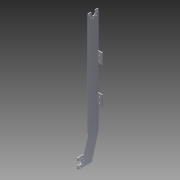
# Autodesk Inventor part: 09
Saved by Autodesk Inventor 2013 (Build 170138000, 138)
## iProperties
Created: 2014-03-10
Part Number: 09
Material: アルミニウム 6061
Document SubType Name: Modeling
Designer: andou
Density: 1 g/cm^3
Author: andou
Title: Dual_Link_Flame(right)
Autodesk Inventor part; units mm, degrees
ref_plane "YZ Plane" through (0, 0, 0) normal (1, 0, 0) x (0, 1, 0)
ref_plane "XZ Plane" through (0, 0, 0) normal (0, 1, 0) x (-1, 0, 0)
ref_plane "XY Plane" through (0, 0, 0) normal (0, 0, 1) x (1, 0, 0)
sketch "スケッチ1" plane through (0, 0, 0) normal (1, 0, 0) x (0, 1, 0)
  line L0 (-20, 125) -> (20, 125)
  line L1 (20, 125) -> (20, -125)
  line L2 (20, -125) -> (-20, -125)
  line L3 (-20, -125) -> (-20, 125)
  point P0 (0, 0)
  dimension "d0" = 250
  dimension "d2" = 40
  dimension "d3" = 20
  dimension "d4" = 125
  constraints: 8 end point, 2 parallel, 1 horizontal, 1 perpendicular
  measures "d0" distance of L2.end L0.start
  measures "d2" distance of L1.end L2.end
  measures "d3" distance from line of L3 point (0, 0)
  measures "d4" distance from line of point (0, 0) L2
extrude "押し出し1" add sketch "スケッチ1" along normal blind 2
sketch "スケッチ3" plane through (0, 0, 0) normal (-1, 0, 0) x (0, 0, 1)
  line L0 (125, -20) -> (125, 20) projected
  line L1 (125, 20) -> (-125, 20) projected
  line L2 (-125, 20) -> (-125, -20) projected
  line L3 (-125, -20) -> (125, -20) projected
  line L4 (-105, -20) -> (-105, -8.0385)
  line L5 (-105, -8.0385) -> (-75, 0)
  line L6 (-75, 0) -> (125, 0)
  line L7 (125, 0) -> (125, 20)
  line L8 (-125, 6.6025) -> (-75, 20)
  point P0 (0, 0)
  dimension "d11" = 20
  dimension "d12" = 15
  dimension "d13" = 15
  dimension "d14" = 20
  dimension "d15" = 250
  dimension "d17" = 200
  dimension "d18" = 200
  constraints: 10 end point, 4 point on line, 3 perpendicular
  measures "d11" distance between parallel lines of L2 L4
  measures "d12" angle of L1 L8
  measures "d13" angle of L6 L5
  measures "d14" distance between parallel lines of L1 L6
  measures "d15" distance between parallel lines of L2 L7
  measures "d17" distance of L7.end L8.end
  measures "d18" distance of L6.end L5.end
extrude "押し出し3" cut sketch "スケッチ3" against normal blind 20 contours L6 L5 L4 L3 L2 L8 L1 L0 keep common part
sketch "スケッチ6" plane through (0, 0, 0) normal (-1, 0, 0) x (0, 0, 1)
  line L0 (-105, -8.0385) -> (-105, -20) projected
  line L1 (-75, 0) -> (-105, -8.0385) projected
  line L2 (125, 0) -> (-75, 0) projected
  line L3 (125, 0) -> (125, 20) projected
  line L4 (125, 20) -> (-75, 20) projected
  line L5 (-125, 6.6025) -> (-75, 20) projected
  line L6 (-125, 6.6025) -> (-125, -20) projected
  line L7 (-125, -20) -> (-105, -20) projected
  arc A0 (-111, -16) -> (-119, -16) centre (-115, -16) ccw
  arc A1 (121, 14) -> (121, 6) centre (121, 10) ccw
  line L8 (-119, -16) -> (-119, -20)
  line L9 (-111, -16) -> (-111, -20)
  line L10 (121, 14) -> (125, 14)
  line L11 (121, 6) -> (125, 6)
  arc A2 (-105.8348, -20) -> (-105, -16) centre (-115, -16) ccw
  arc A3 (-125, -16) -> (-124.1652, -20) centre (-115, -16) ccw
  arc A4 (121, 0) -> (125, 0.8348) centre (121, 10) ccw
  arc A5 (125, 19.1652) -> (121, 20) centre (121, 10) ccw
  point P0 (0, 0)
  dimension "d37" = 8
  dimension "d39" = 8
  dimension "d40" = 4
  dimension "d41" = 4
  dimension "d42" = 10
  dimension "d43" = 10
  constraints: 12 point on circle, 12 point on line, 8 end point, 6 centre point, 6 tangent, 3 perpendicular, 2 coincident, 2 concentric, 1 parallel
  measures "d37" diameter of A0
  measures "d39" diameter of A1
  measures "d40" distance from line of A0.centre L7
  measures "d41" distance from line of A1.centre L3
  measures "d42" distance from line of L4 A1.centre
  measures "d43" distance from line of L6 A0.centre
extrude "押し出し6" cut sketch "スケッチ6" against normal blind 11 contours L0 A2 L7 L9 A0 L8 A3 L6 L5 L4 A5 L3 L10 A1 L11 A4 L2 L1 keep common part
sketch "スケッチ7" plane through (0, 0, 0) normal (-1, 0, 0) x (0, 0, 1)
  arc A0 (125, 19.1652) -> (121, 20) centre (121, 10) ccw projected
  arc A1 (-125, -16) -> (-124.1652, -20) centre (-115, -16) ccw projected
  line L0 (-124.1652, -20) -> (-119, -20) projected
  line L1 (125, 0.8348) -> (125, 6) projected
  circle A2 centre (121, 3) radius 1
  circle A3 centre (-122, -16) radius 1
  point P0 (0, 0)
  dimension "d46" = 2
  dimension "d48" = 7
  dimension "d49" = 4
  dimension "d50" = 4
  dimension "d51" = 7
  constraints: 2 centre point, 1 equal radius
  measures "d46" diameter of A2
  measures "d48" distance of A0.centre A2.centre
  measures "d49" distance from line of L1 A2.centre
  measures "d50" distance from line of A3.centre L0
  measures "d51" distance of A1.centre A3.centre
hole "穴1" at (0, -16, -122) at (0, 3, 121) direction (1, 0, 0) diameter 2 end through all
pattern_circular "円形状パターン1" count 5 over 180 about axis through (0, -16, -115) along (1, 0, 0) of "穴1"
pattern_circular "円形状パターン2" count 5 over 180 about axis through (0, 10, 121) along (1, 0, 0) of "穴1"
sketch "スケッチ12" plane through (2, 0, 0) normal (1, 0, 0) x (0, 0, -1)
  line L0 (-125, 19.1652) -> (-125, 14) projected
  line L1 (75, 20) -> (-121, 20) projected
  line L2 (35, 20) -> (15, 20)
  line L3 (15, 20) -> (15, 18)
  line L4 (15, 18) -> (35, 18)
  line L5 (35, 18) -> (35, 20)
  line L6 (-35, 20) -> (-55, 20)
  line L7 (-55, 20) -> (-55, 18)
  line L8 (-55, 18) -> (-35, 18)
  line L9 (-35, 18) -> (-35, 20)
  point P0 (0, 0)
  dimension "d96" = 2
  dimension "d98" = 20
  dimension "d99" = 140
  dimension "d120" = 50
  constraints: 16 end point, 4 parallel, 2 equal length, 2 horizontal, 2 perpendicular, 2 point on line
  measures "d96" distance between parallel lines of L2 L4
  measures "d98" distance between parallel lines of L5 L3
  measures "d99" distance between parallel lines of L0 L3
  measures "d120" distance between parallel lines of L3 L9
extrude "押し出し11" add sketch "スケッチ12" along normal blind 8
sketch "スケッチ14" plane through (0, 20, 121) normal (0, 1, 0) x (1, 0, 0)
  line L0 (10, 86) -> (10, 66) projected
  line L1 (2, 86) -> (10, 86) projected
  line L2 (10, 156) -> (10, 136) projected
  line L3 (2, 156) -> (10, 156) projected
  circle A0 centre (5, 81) radius 1.3
  circle A1 centre (5, 71) radius 1.3
  circle A2 centre (5, 141) radius 1.3
  circle A3 centre (5, 151) radius 1.3
  point P0 (0, 121)
  dimension "d123" = 5
  dimension "d124" = 5
  dimension "d125" = 5
  dimension "d126" = 5
  dimension "d127" = 2.6
  dimension "d128" = 10
  dimension "d129" = 10
  dimension "d130" = 5
  dimension "d131" = 5
  constraints: 4 centre point, 3 equal radius
  measures "d123" distance from line of L0 A0.centre
  measures "d124" distance from line of L0 A1.centre
  measures "d125" distance from line of A2.centre L2
  measures "d126" distance from line of A3.centre L2
  measures "d127" diameter of A3
  measures "d128" distance of A3.centre A2.centre
  measures "d129" distance of A1.centre A0.centre
  measures "d130" distance from line of L1 A0.centre
  measures "d131" distance from line of L3 A3.centre
hole "穴4" at (5, 20, 50) at (5, 20, -20) at (5, 20, -30) at (5, 20, 40) direction (0, -1, 0) diameter 2.6 depth 2 tip angle 118
